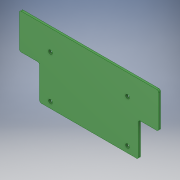
# Autodesk Inventor part: PCBPuissance
Saved by Autodesk Inventor 2019 (Build 230136000, 136)
## iProperties
Created: 2019-07-30
Part Number: PCBPuissance
Material: Résine phénolique
Document SubType Name: Modeling
Designer: Sébastien DI MERCURIO
Density: 1.38 g/cm^3
Appearance: Lisse - Vert forêt foncé
Author: Sébastien DI MERCURIO
Autodesk Inventor part; units mm, degrees
ref_plane "YZ Plane" through (0, 0, 0) normal (1, 0, 0) x (0, 1, 0)
ref_plane "XZ Plane" through (0, 0, 0) normal (0, 1, 0) x (-1, 0, 0)
ref_plane "XY Plane" through (0, 0, 0) normal (0, 0, 1) x (1, 0, 0)
sketch "Esquisse1" plane through (0, 0, 0) normal (0, 0, 1) x (1, 0, 0)
  line L0 (0, 0) -> (114, 0)
  line L1 (114, 0) -> (114, 57)
  line L2 (114, 57) -> (0, 57)
  line L3 (0, 57) -> (0, 0)
  dimension "d0" = 114
  dimension "d1" = 57
  constraints: 8 end point, 2 parallel, 1 horizontal, 1 perpendicular
  measures "d0" distance of L1.end L2.end
  measures "d1" distance of L0.end L1.end
extrude "Extrusion1" add sketch "Esquisse1" along normal blind 1.6
sketch "Esquisse2" plane through (0, 0, 1.6) normal (0, 0, 1) x (1, 0, 0)
  line L0 (0, 0) -> (16.5, 0)
  line L1 (16.5, 0) -> (16.5, 28)
  line L2 (16.5, 28) -> (0, 28)
  line L3 (0, 28) -> (0, 0)
  line L4 (114, 0) -> (97.5, 0)
  line L5 (97.5, 0) -> (97.5, 28)
  line L6 (97.5, 28) -> (114, 28)
  line L7 (114, 28) -> (114, 0)
  dimension "d5" = 28
  dimension "d9" = 81
  constraints: 16 end point, 4 parallel, 2 horizontal, 2 perpendicular, 2 point on line, 1 collinear
  measures "d5" distance of L2.end L0.start
  measures "d9" distance of L4.end L0.end
extrude "Extrusion2" cut sketch "Esquisse2" against normal through all
fillet "Congé1" radius 1.5 8 edges at (0, 57, 0.8) (0, 28, 0.8) (16.5, 0, 0.8) (16.5, 28, 0.8) (97.5, 28, 0.8) (97.5, 0, 0.8) (114, 28, 0.8) (114, 57, 0.8)
sketch "Esquisse3" plane through (0, 0, 1.6) normal (0, 0, 1) x (1, 0, 0)
  circle A0 centre (25.5, 5) radius 1.6
  circle A1 centre (88.5, 5) radius 1.6
  circle A2 centre (88.5, 40) radius 1.6
  circle A3 centre (25.5, 40) radius 1.6
  line L0 (97.5, 1.5) -> (97.5, 26.5) projected
  line L1 (16.5, 26.5) -> (16.5, 1.5) projected
  line L2 (18, 0) -> (96, 0) projected
  point P0 (0, 0)
  dimension "d10" = 63
  dimension "d11" = 81
  dimension "d12" = 9
  dimension "d13" = 35
  dimension "d14" = 5
  dimension "d15" = 3.2
  constraints: 4 centre point, 3 equal radius, 2 horizontal alignment, 2 vertical alignment
  measures "d10" distance of A1.centre A0.centre
  measures "d11" distance between parallel lines of L0 L1
  measures "d12" distance from line of L1 A0.centre
  measures "d13" distance of A0.centre A3.centre
  measures "d14" distance from line of L2 A0.centre
  measures "d15" diameter of A3
extrude "Extrusion3" cut sketch "Esquisse3" against normal through all
equation "\"d12\" = -0.5 * d10 + 0.5 * d11"
